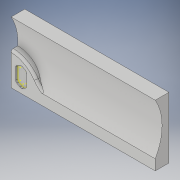
# Autodesk Inventor part: prototype #1
Saved by Autodesk Inventor 2018 (Build 220112000, 112)
## iProperties
Created: 2017-11-02
Part Number: prototype #1
Material: Generic
Document SubType Name: Modeling
Designer: 990813
Density: 1 g/cm^3
Appearance: Default
Author: 990813
Autodesk Inventor part; units mm, degrees
ref_plane "YZ Plane" through (0, 0, 0) normal (1, 0, 0) x (0, 1, 0)
ref_plane "XZ Plane" through (0, 0, 0) normal (0, 1, 0) x (-1, 0, 0)
ref_plane "XY Plane" through (0, 0, 0) normal (0, 0, 1) x (1, 0, 0)
sketch "Sketch1" plane through (0, 0, 0) normal (0, 0, 1) x (1, 0, 0)
  line L0 (0, 0) -> (200, 0)
  line L1 (200, 0) -> (200, 85)
  line L2 (200, 85) -> (0, 85)
  line L3 (0, 85) -> (0, 0)
  dimension "d0" = 200
  dimension "d1" = 85
  constraints: 8 end point, 2 parallel, 1 horizontal, 1 perpendicular
  measures "d0" distance of L2.end L1.end
  measures "d1" distance of L1.end L0.end
extrude "Extrusion1" add sketch "Sketch1" along normal blind 19
sketch "Sketch2" plane through (200, 0, 0) normal (1, 0, 0) x (0, 0, -1)
  line L0 (0, 0) -> (-19, 0) projected
  line L1 (0, 85) -> (-19, 85) projected
  line L2 (-19, 0) -> (-19, 14.605)
  line L3 (-19, 0) -> (-19, 85) projected
  arc A0 (-19, 14.605) -> (-19, 85) centre (-79.4534, 49.8025) ccw
  dimension "d9" = 14.605
  constraints: 2 end point, 2 point on circle, 1 centre point, 1 point on line
  measures "d9" distance of L0.end L2.end
extrude "Extrusion2" cut sketch "Sketch2" against normal through all
sketch "Sketch9" plane through (0, 0, 19) normal (0, 0, 1) x (1, 0, 0)
  line L0 (200, 14.605) -> (0, 14.605) projected
  line L1 (0, 14.605) -> (0, 85) projected
  arc A0 (40.2378, 14.605) -> (0, 45.6428) centre (-0.879, 2.9021) ccw
  line L2 (0, 45.6428) -> (0, 14.605)
  line L3 (49.8468, 14.605) -> (0, 14.605)
  arc A1 (34.584, 26.7752) -> (49.8468, 14.605) centre (58.9671, 41.6987) ccw
  point P0 (0, 0)
  point P1 (38.109, 20.4373)
  constraints: 6 point on circle, 4 end point, 3 point on line, 2 centre point, 2 collinear
extrude "Extrusion6" add sketch "Sketch9" against normal blind 12.7 contours L0 A0 A1 | L0 L1 A0 A1
fillet "Fillet4" radius 3.175 2 edges at (19.5949, 40.4303, 19) (41.1444, 19.347, 19)
sketch "Sketch10" plane through (0, 0, 19) normal (0, 0, 1) x (1, 0, 0)
  line L0 (21.6079, 10.4672) -> (13.9879, 6.0678)
  line L1 (13.9879, 6.0678) -> (6.3679, 10.4672)
  line L2 (6.3679, 29.8109) -> (13.9879, 34.2103)
  line L3 (13.9879, 34.2103) -> (21.6079, 29.8109)
  line L4 (6.3679, 29.8109) -> (6.3679, 10.4672)
  line L5 (21.6079, 29.8109) -> (21.6079, 10.4672)
  point P0 (0, 0)
  point P1 (13.9879, 20.1391)
  dimension "d24" = 28.1426
  dimension "d29" = 15.24
  dimension "d30" = 4.3994
  constraints: 12 end point, 1 vertical, 3 other
  measures "d24" distance of L0.end L2.end
  measures "d29" distance between parallel lines of L5 L4
  measures "d30" vertical distance of L1.end L0.end
extrude "Extrusion7" cut sketch "Sketch10" against normal blind 3
fillet "Fillet5" radius 3.302 6 edges at (13.9879, 34.2103, 17.5) (21.6079, 29.8109, 17.5) (6.3679, 29.8109, 17.5) (6.3679, 10.4672, 17.5) (13.9879, 6.0678, 17.5) (21.6079, 10.4672, 17.5)
sketch "Sketch11" plane through (0, 0, 16) normal (0, 0, 1) x (1, 0, 0)
  arc A0 (19.9569, 9.514) -> (21.6079, 12.3736) centre (18.3059, 12.3736) ccw projected
  line L0 (21.6079, 27.9045) -> (21.6079, 12.3736) projected
  arc A1 (21.6079, 27.9045) -> (19.9569, 30.7641) centre (18.3059, 27.9045) ccw projected
  line L1 (15.6389, 33.2571) -> (19.9569, 30.7641) projected
  arc A2 (15.6389, 33.2571) -> (12.3369, 33.2571) centre (13.9879, 30.3975) ccw projected
  line L2 (8.0189, 30.7641) -> (12.3369, 33.2571) projected
  arc A3 (8.0189, 30.7641) -> (6.3679, 27.9045) centre (9.6699, 27.9045) ccw projected
  line L3 (6.3679, 12.3736) -> (6.3679, 27.9045) projected
  arc A4 (6.3679, 12.3736) -> (8.0189, 9.514) centre (9.6699, 12.3736) ccw projected
  line L4 (12.3369, 7.021) -> (8.0189, 9.514) projected
  arc A5 (12.3369, 7.021) -> (15.6389, 7.021) centre (13.9879, 9.8806) ccw projected
  line L5 (19.9569, 9.514) -> (15.6389, 7.021) projected
  point P0 (0, 0)
body "Solid1"
